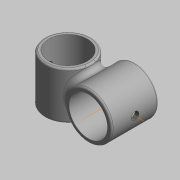
# Autodesk Inventor part: L45-7
Saved by Autodesk Inventor 2019.4 (Build 234330000, 330)
## iProperties
Created: 2020-04-23
Part Number: L45-7
Material: Generic
Document SubType Name: Modeling
Designer: Hannah
Density: 1 g/cm^3
Appearance: Default
Author: Hannah
Autodesk Inventor part; units mm, degrees
ref_plane "XZ Plane" through (0, 0, 0) normal (0, 1, 0) x (-1, 0, 0)
ref_plane "XY Plane" through (0, 0, 0) normal (0, 0, 1) x (1, 0, 0)
sketch "Sketch1" plane through (0, 0, 0) normal (0, 0, 1) x (1, 0, 0)
  circle A0 centre (0, 0) radius 22
  circle A1 centre (0, 0) radius 26.5
  dimension "d1" = 53
  dimension "d2" = 44
  constraints: 2 centre point, 2 coincident
  measures "d1" diameter of A1
  measures "d2" diameter of A0
extrude "Extrusion1" add sketch "Sketch1" along normal mid plane 54 contours A0 | A1
sketch "Sketch2" plane through (0, 0, 0) normal (0, 1, 0) x (-1, 0, 0)
  circle A0 centre (50, 0) radius 22
  circle A1 centre (50, 0) radius 26.5
  line L0 (91.8, 0) -> (-15.3, 0) projected
  line L1 (0, -37.1) -> (0, 37.1) projected
  point P0 (0, 0)
  dimension "d5" = 44
  dimension "d6" = 53
  dimension "d13" = 50
  constraints: 2 centre point, 1 coincident, 1 point on line
  measures "d5" diameter of A0
  measures "d6" diameter of A1
  measures "d13" distance from line of L1 A0.centre
extrude "Extrusion2" add sketch "Sketch2" along normal mid plane 54
fillet "Fillet1" radius 5 4 edges at (-24.9999, 8.7894, 8.789) (-25, 8.7892, -8.7892) (-25, -8.7892, -8.7892) (-25, -8.7892, 8.7892)
extrude "Extrusion3" cut sketch "Sketch2" along normal through all both and the other way through all contours L0 A0 | A0 L0
extrude "Extrusion4" cut sketch "Sketch1" along normal through all both and the other way through all contours A0
hole "Hole1" at (0, 0, 0) direction (1, 0, 0) diameter 8.917 end through all thread size "M10x1" class "6H" standard "ISO Metric profile"
ref_plane "Work Plane1" through (-50, 0, 0) normal (1, 0, 0) x (0, 1, 0)
hole "Hole2" at (-50, 0, 0) direction (-1, 0, 0) diameter 8.917 end through all thread size "M10x1" class "6H" standard "ISO Metric profile"
fillet "Fillet2" radius 2 4 edges at (-23.5, 27, 0) (-23.5, -27, 0) (-26.5, 0, 27) (-26.5, 0, -27)
equation "\"d5\" = d2"
equation "\"d6\" = d1"
equation "\"d7\" = d3"
equation "\"d3\" = 54"
body "Solid1"
